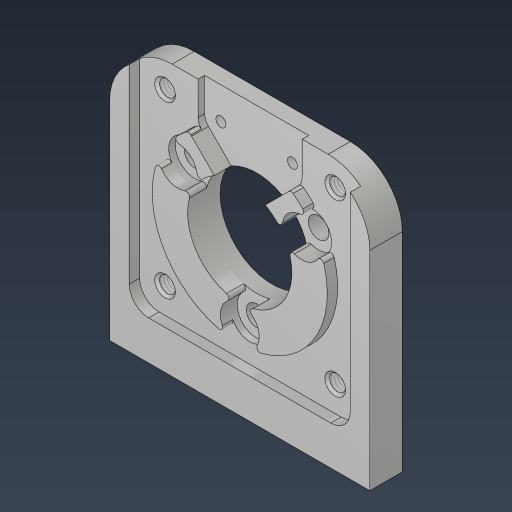
# Autodesk Inventor part: Lagerbock Getriebe
Saved by Autodesk Inventor 2023.1 (Build 271208000, 208)
## iProperties
Part Number: Lagerbock Getriebe
Material: Aluminium 6061
Document SubType Name: Modeling
Designer: rYan
Density: 2.7 g/cm^3
Appearance: Aluminium - flach
Mass: 15.0828 g
Surface Area: 41.0098 cm^2
Volume: 5.5862 cm^3
Author: rYan
Autodesk Inventor part; units mm, degrees
ref_plane "YZ Plane" through (0, 0, 0) normal (1, 0, 0) x (0, 1, 0)
ref_plane "XZ Plane" through (0, 0, 0) normal (0, 1, 0) x (-1, 0, 0)
ref_plane "XY Plane" through (0, 0, 0) normal (0, 0, 1) x (1, 0, 0)
sketch "Skizze1" plane through (0, 0, 0) normal (0, 1, 0) x (-1, 0, 0)
  line L0 (20, 0) -> (-20, 0)
  line L1 (-20, 0) -> (-20, 40)
  line L2 (-20, 40) -> (20, 40)
  line L3 (20, 40) -> (20, 0)
  line L4 (0, -9) -> (0, 54) construction
  circle A0 centre (0, 23) radius 0.5
  circle A1 centre (0, 23) radius 22 construction
  line L5 (22, 23) -> (-22, 23) construction
  point P0 (0, 0)
  dimension "d0" = 40
  dimension "d1" = 40
  dimension "d83" = 1
  dimension "d85" = 44
  dimension "d176" = 23
  constraints: 10 end point, 3 midpoint, 2 centre point, 2 horizontal, 2 parallel, 2 point on circle, 1 coincident, 1 perpendicular, 1 point on line, 1 other
  measures "d0" distance of L2.end L0.start
  measures "d1" distance of L1.end L2.end
  measures "d83" diameter of A0
  measures "d85" diameter of A1
  measures "d176" distance between parallel lines of L0 L5
extrude "Extrusion1" add sketch "Skizze1" along normal mid plane 5
sketch "Skizze12" plane through (0, -2.5, 0) normal (0, -1, 0) x (1, 0, 0)
  circle A0 centre (0, 23) radius 0.5 projected
  circle A1 centre (0, 23) radius 0.5 projected
  point P0 (0, 0)
  constraints: 1 coincident
hole "Motormitte" at (0, -2.5, 23) direction (0, 1, 0) diameter 16.04 end through all
sketch "Skizze13" plane through (0, -2.5, 0) normal (0, -1, 0) x (1, 0, 0)
  circle A0 centre (0, 23) radius 0.5 projected
  circle A1 centre (0, 23) radius 0.5 construction
  circle A2 centre (0, 23) radius 11 construction
  line L0 (0, 23) -> (0, 12) construction
  point P0 (0, 0)
  dimension "d106" = 22
  constraints: 2 coincident, 2 end point, 1 vertical, 1 vertical alignment, 2 other
hole "Motorschraube" at (0, -2.5, 12) direction (0, 1, 0) diameter 3.2 end through all counterbore diameter 6 counterbore depth 2.6
pattern_circular "Motorschrauben" count 3 over 360 about axis through (0, 54.2891, 23) along (0, -1, 0) of "Motorschraube"
sketch "Skizze14" plane through (20, 2.5, 0) normal (0, 0, -1) x (-1, 0, 0)
  line L0 (20, -6) -> (20, 1) projected
  line L1 (12.9116, -5) -> (27.0884, -5) projected
  line L2 (28.02, 0) -> (28.02, 0) projected
  line L3 (20, -5) -> (20, 0) construction
  line L4 (32, -2.5) -> (8, -2.5) construction
  line L5 (23, -5) -> (17, -5) projected
  line L6 (40, 0) -> (40, -5) projected
  line L7 (0, 0) -> (40, 0) projected
  line L8 (0, 0) -> (0, -5) projected
  line L9 (40, -5) -> (0, -5) projected
  point P0 (20, -2.5)
  point P1 (20, -2.5)
  point P2 (19.7048, -5)
  point P3 (20.2952, -5)
  point P4 (20, -2.5)
  dimension "d139" = 24
  constraints: 4 end point, 4 midpoint, 1 coincident, 1 horizontal
  measures "d139" distance of L4.start L4.end
hole "Montage" at (-12, 0, 0) at (12, 0, 0) at (0, 0, 0) direction (0, 0, 1) diameter 2.459 depth 4.5 tip angle 118 thread size "M3x0.5" class "6H" standard "ISO Metric profile"
fillet "Rundung1" radius 8 2 edges at (20, 0, 40) (-20, 0, 40)
sketch "Skizze21" plane through (0, -2.5, 0) normal (0, -1, 0) x (1, 0, 0)
  arc A0 (6.7932, 27.263) -> (-0.2952, 14.9854) centre (0, 23) ccw projected
  circle A1 centre (0, 23) radius 13.46
  line L0 (-17, 40) -> (17, 40)
  line L1 (17, 40) -> (17, 6)
  line L2 (17, 6) -> (-17, 6)
  line L3 (-17, 6) -> (-17, 40)
  line L4 (-17, 40) -> (17, 6) construction
  line L5 (17, 40) -> (-17, 6) construction
  point P0 (0, 0)
  dimension "d177" = 26.92
  dimension "d224" = 34
  dimension "d225" = 34
  constraints: 12 end point, 2 coincident, 2 parallel, 1 centre point, 1 horizontal, 1 midpoint, 1 perpendicular
  measures "d177" diameter of A1
  measures "d224" distance of L1.end L2.end
  measures "d225" distance of L0.end L1.end
extrude "Extrusion8" cut sketch "Skizze21" against normal blind 1.6
fillet "Rundung3" radius 3 2 edges at (17, -1.7, 6) (-17, -1.7, 6)
sketch "Skizze22" plane through (0, -2.5, 23) normal (0, -1, 0) x (1, 0, 0)
  circle A0 centre (-5.5, 12.0859) radius 2 construction
  circle A1 centre (5.5, 12.0859) radius 2 construction
  line L0 (-2.0788, 13.9499) -> (1.9212, 13.9499) construction
  line L1 (1.9212, 13.9499) -> (1.9212, 8.7499) construction
  line L2 (1.9212, 8.7499) -> (-2.0788, 8.7499) construction
  line L3 (-2.0788, 8.7499) -> (-2.0788, 13.9499) construction
  line L4 (-8, 11.0859) -> (-3.9141, 7)
  line L5 (-3.9141, 7) -> (3.9141, 7)
  line L6 (3.9141, 7) -> (8, 11.0859)
  line L7 (8, 11.0859) -> (8, 17)
  line L8 (8, 17) -> (-8, 17)
  line L9 (-8, 17) -> (-8, 11.0859)
  arc A2 (0.2952, -8.0146) -> (-6.7932, 4.263) centre (0, 0) ccw construction
  line L10 (0, 0) -> (0, 17) construction
  line L11 (-12, 17) -> (12, 17) construction
  circle A3 centre (0, 0) radius 12.7 construction
  line L12 (-2.0788, 11.3499) -> (1.9212, 11.3499) construction
  circle A4 centre (0, 0) radius 10.2 construction
  arc A5 (-7.0884, 3.7516) -> (7.0884, 3.7516) centre (0, 0) ccw construction
  line L13 (-8, 11.0859) -> (8, 11.0859) construction
  point P0 (0, -23)
  dimension "d181" = 4
  dimension "d182" = 4
  dimension "d183" = 5.2
  dimension "d184" = 4
  dimension "d185" = 25.4
  dimension "d186" = 20.4
  dimension "d187" = 45
  dimension "d188" = 7
  dimension "d189" = 16
  dimension "d192" = 11
  dimension "d193" = 1
  constraints: 27 end point, 4 centre point, 3 horizontal, 3 midpoint, 3 perpendicular, 2 coincident, 2 parallel, 1 collinear, 1 point on circle, 1 symmetric about line, 2 other
  measures "d181" diameter of A0
  measures "d182" diameter of A1
  measures "d183" distance of L0.end L1.end
  measures "d184" distance of L0.start L0.end
  measures "d185" diameter of A3
  measures "d186" diameter of A4
  measures "d187" angle of L4 L5
  measures "d188" distance from line of A3.centre L5
  measures "d189" distance of L7.end L8.end
  measures "d192" distance of A1.centre A0.centre
  measures "d193" distance from line of L13 A1.centre
extrude "Extrusion9" cut sketch "Skizze22" against normal blind 2.6
sketch "Skizze23" plane through (0, 0.1, 23) normal (0, -1, 0) x (1, 0, 0)
  arc A0 (3.9141, 7) -> (-3.9141, 7) centre (0, 0) ccw projected
  line L0 (8, 11.0859) -> (3.9141, 7) projected
  line L1 (8, 17) -> (8, 11.0859) projected
  line L2 (-8, 17) -> (8, 17) projected
  line L3 (-8, 11.0859) -> (-8, 17) projected
  line L4 (-3.9141, 7) -> (-8, 11.0859) projected
  line L5 (-8, 11.0859) -> (-8, 17) construction
  line L6 (-8, 11.0859) -> (8, 11.0859) construction
  line L7 (0, 0) -> (0, 17) construction
  line L8 (-12, 17) -> (12, 17) construction
  point P0 (0, -23)
  point P1 (-5.5, 12.0859)
  point P2 (5.5, 12.0859)
  dimension "d194" = 11
  dimension "d195" = 1
  constraints: 4 end point, 1 midpoint, 1 perpendicular, 1 symmetric about line
  measures "d194" distance of point (5.5, 12.086) point (-5.5, 12.086)
  measures "d195" distance from line of L6 point (5.5, 12.086)
hole "Bohrung13" at (-5.5, 0.1, 35.0859) at (5.5, 0.1, 35.0859) direction (0, 1, 0) diameter 1.567 end through all thread size "M2x0.4" class "6H" standard "ISO Metric profile"
fillet "Rundung2" radius 2 2 edges at (-8, -0.4, 34.0859) (8, -0.4, 34.0859)
sketch "Skizze26" plane through (0, -0.9, 0) normal (0, -1, 0) x (1, 0, 0)
  circle A0 centre (0, 23) radius 8.02 construction
  circle A1 centre (0, 23) radius 18.5
  line L0 (-13.0815, 36.0815) -> (13.0815, 9.9185) construction
  line L1 (-13.0815, 9.9185) -> (13.0815, 36.0815) construction
  line L2 (0, 50.4) -> (0, -8.4) construction
  point P0 (0, 0)
  dimension "d216" = 37
  constraints: 5 coincident, 4 end point, 4 point on circle, 3 midpoint, 1 centre point, 1 perpendicular, 1 other
  measures "d216" diameter of A1
hole "Bohrung14" at (-13.0815, -0.9, 36.0815) at (13.0815, -0.9, 36.0815) at (13.0815, -0.9, 9.9185) at (-13.0815, -0.9, 9.9185) direction (0, 1, 0) diameter 2.459 end through all countersink diameter 3.2 countersink angle 90 thread size "M3x0.5" class "6H" standard "ISO Metric profile"
sketch "Skizze27" plane through (0, -0.9, 0) normal (0, -1, 0) x (1, 0, 0)
  line L0 (8, 40) -> (12, 40) projected
  line L1 (-17, 9) -> (-17, 38.245) projected
  line L2 (17, 38.245) -> (17, 9) projected
  line L3 (-17, 38.245) -> (-17, 42)
  line L4 (-17, 42) -> (17, 42)
  line L5 (17, 42) -> (17, 38.245)
  line L6 (7.4142, 33.5001) -> (3.9141, 30) projected
  arc A0 (7.4142, 33.5001) -> (7.773, 33.9888) centre (6, 34.9143) ccw projected
  line L7 (-3.9141, 30) -> (-7.4142, 33.5001) projected
  arc A1 (-7.773, 33.9888) -> (-7.4142, 33.5001) centre (-6, 34.9143) ccw projected
  arc A2 (-7.773, 33.9888) -> (7.773, 33.9888) centre (0, 23) ccw projected
  arc A3 (3.9141, 30) -> (-3.9141, 30) centre (0, 23) ccw construction
  arc A4 (14, 6) -> (17, 9) centre (14, 9) ccw projected
  line L8 (14, 6) -> (-14, 6) projected
  arc A5 (-17, 9) -> (-14, 6) centre (-14, 9) ccw projected
  arc A6 (2.4244, 28.5102) -> (-2.4244, 28.5102) centre (0, 23) ccw
  line L9 (3.9141, 30) -> (2.4244, 28.5102)
  line L10 (-3.9141, 30) -> (-2.4244, 28.5102)
  point P0 (0, 0)
  dimension "d228" = 2
  dimension "d229" = 2
  constraints: 10 end point, 3 collinear, 2 point on circle, 1 centre point, 1 coincident, 1 perpendicular, 1 vertical
  measures "d228" distance between parallel lines of L4 L0
  measures "d229" radial gap between concentric circles of A3 A6
sketch "Skizze28" plane through (0, 0.1, 23) normal (0, -1, 0) x (1, 0, 0)
  arc A0 (2.4244, 5.5102) -> (-2.4244, 5.5102) centre (0, 0) ccw projected
  line L0 (3.9141, 7) -> (2.4244, 5.5102) projected
  line L1 (-3.9141, 7) -> (-2.4244, 5.5102) projected
  line L2 (-3.9141, 7) -> (-7.4142, 10.5001) projected
  line L3 (7.4142, 10.5001) -> (3.9141, 7) projected
  arc A1 (7.4142, 10.5001) -> (7.773, 10.9888) centre (6, 11.9143) ccw projected
  arc A2 (-7.773, 10.9888) -> (-7.4142, 10.5001) centre (-6, 11.9143) ccw projected
  arc A3 (-8, 11.9143) -> (-7.773, 10.9888) centre (-6, 11.9143) ccw projected
  line L4 (-8, 11.9143) -> (-8, 17) projected
  arc A4 (7.773, 10.9888) -> (8, 11.9143) centre (6, 11.9143) ccw projected
  line L5 (8, 17) -> (8, 11.9143) projected
  line L6 (8, 17) -> (8, 19)
  line L7 (8, 19) -> (-8, 19)
  line L8 (-8, 19) -> (-8, 17)
  point P0 (0, -23)
  dimension "d230" = 2
  constraints: 6 end point, 2 perpendicular, 1 vertical
  measures "d230" distance from line of L5.start L7
fillet "Rundung4" radius 0.5 14 edges at (0.2952, -1.2, 14.9854) (-0.2952, -1.2, 14.9854) (-1.8947, -1.7, 9.674) (1.8947, -1.7, 9.674) (-7.0884, -1.2, 26.7516) (-6.7932, -1.2, 27.263) (-10.5933, -1.7, 31.3038) (-12.488, -1.7, 28.0222) (6.7932, -1.2, 27.263) (7.0884, -1.2, 26.7516) (12.488, -1.7, 28.0222) (10.5933, -1.7, 31.3038) (7.773, -1.7, 33.9888) (-7.773, -1.7, 33.9888)
